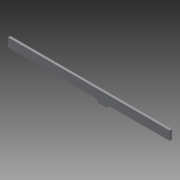
# Autodesk Inventor part: Granny Gearbox Routing Template Horizontal Tabs
Saved by Autodesk Inventor 2015 (Build 190159000, 159)
## iProperties
Created: 2016-02-25
Part Number: Granny Gearbox Routing Template Horizontal Tabs
Material: Generic
Document SubType Name: Modeling
Designer: sethbattis
Density: 1 g/cm^3
Appearance: Default
Author: sethbattis
Autodesk Inventor part; units mm, degrees
ref_plane "YZ Plane" through (0, 0, 0) normal (1, 0, 0) x (0, 1, 0)
ref_plane "XZ Plane" through (0, 0, 0) normal (0, 1, 0) x (-1, 0, 0)
ref_plane "XY Plane" through (0, 0, 0) normal (0, 0, 1) x (1, 0, 0)
sketch "Sketch1" plane through (0, 0, 0) normal (0, 0, 1) x (1, 0, 0)
  line L0 (-86.188, -1.6122) -> (142.412, -1.6122)
  line L1 (142.412, -1.6122) -> (142.412, -14.3122)
  line L2 (142.412, -14.3122) -> (57.4807, -14.3122)
  line L3 (-86.188, -14.3122) -> (-86.188, -1.6122)
  line L4 (53.512, -18.2809) -> (53.512, -18.2809)
  line L5 (53.512, -18.2809) -> (40.812, -18.2809)
  line L6 (40.812, -18.2809) -> (40.812, -18.2809)
  line L7 (36.8432, -14.3122) -> (-86.188, -14.3122)
  arc A0 (40.812, -18.2809) -> (36.8432, -14.3122) centre (36.8432, -18.2809) ccw
  arc A1 (57.4807, -14.3122) -> (53.512, -18.2809) centre (57.4807, -18.2809) ccw
  point P0 (0, 0)
  point P1 (53.512, -14.3122)
  dimension "d0" = 228.6
  dimension "d1" = 12.7
  dimension "d2" = 12.7
  dimension "d3" = 3.9688
  dimension "d4" = 88.9
  dimension "d5" = 3.9688
  constraints: 16 end point, 4 parallel, 4 point on circle, 4 tangent, 2 centre point, 2 point on line, 1 equal radius, 1 horizontal, 1 perpendicular
  measures "d0" distance of L1.end L3.start
  measures "d1" distance of L0.end L1.end
  measures "d2" distance of L4.end L5.end
  measures "d3" distance of point (53.512, -14.312) L4.end
  measures "d4" distance between parallel lines of L1 L4
  measures "d5" radius of A0
extrude "Extrusion1" add sketch "Sketch1" along normal blind 3.175
body "Solid1"
